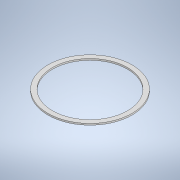
# Autodesk Inventor part: 65. Кольцо упорное подшипника
Saved by Autodesk Inventor 2021 (Build 250183000, 183)
## iProperties
Created: 2021-03-10
Part Number: 65. Кольцо упорное подшипника
Material: Типовые
Document SubType Name: Modeling
Designer: Данил
Density: 1 g/cm^3
Appearance: По умолчанию
Author: Данил
Autodesk Inventor part; units mm, degrees
ref_plane "YZ Plane" through (0, 0, 0) normal (1, 0, 0) x (0, 1, 0)
ref_plane "XZ Plane" through (0, 0, 0) normal (0, 1, 0) x (-1, 0, 0)
ref_plane "XY Plane" through (0, 0, 0) normal (0, 0, 1) x (1, 0, 0)
sketch "Эскиз1" plane through (0, 0, 0) normal (0, 0, 1) x (1, 0, 0)
  line L0 (0, 0.85) -> (0, -0.85)
  line L1 (40.5, 0.85) -> (40.5, -0.85)
  line L2 (40.5, -0.85) -> (45.4, -0.85)
  line L3 (45.4, -0.85) -> (45.4, 0.85)
  line L4 (45.4, 0.85) -> (40.5, 0.85)
  point P0 (0, 0)
  point P1 (0, 0)
  dimension "d0" = 1.7
  dimension "d1" = 81
  dimension "d2" = 4.9
  constraints: 10 end point, 3 perpendicular, 2 horizontal alignment, 2 vertical, 1 coincident, 1 midpoint
  measures "d0" distance of L0.start L0.end
  measures "d1" diameter of L1 L0
  measures "d2" distance between parallel lines of L3 L1
revolve "Вращение1" add sketch "Эскиз1" angle 360 about axis through (0, 0.85, 0) along (0, -1, 0)
